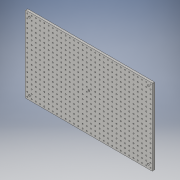
# Autodesk Inventor part: MB1830_solid
Saved by Autodesk Inventor 2016 (Build 200138000, 138)
## iProperties
Created: 2018-01-13
Part Number: MB1830_solid
Material: Generic
Document SubType Name: Modeling
Designer: harveylab
Density: 1 g/cm^3
Appearance: Default
Author: harveylab
Autodesk Inventor part; units mm, degrees
ref_plane "YZ Plane" through (0, 0, 0) normal (1, 0, 0) x (0, 1, 0)
ref_plane "XZ Plane" through (0, 0, 0) normal (0, 1, 0) x (-1, 0, 0)
ref_plane "XY Plane" through (0, 0, 0) normal (0, 0, 1) x (1, 0, 0)
sketch "Sketch1" plane through (0, 0, 0) normal (0, 0, 1) x (1, 0, 0)
  line L0 (-2.7, 453.9) -> (-2.7, 2.7)
  arc A0 (-2.7, 2.7) -> (0, 0) centre (0, 2.7) ccw
  line L1 (0, 0) -> (756, 0)
  arc A1 (756, 0) -> (758.7, 2.7) centre (756, 2.7) ccw
  line L2 (758.7, 2.7) -> (758.7, 453.9)
  arc A2 (758.7, 453.9) -> (756, 456.6) centre (756, 453.9) ccw
  line L3 (756, 456.6) -> (0, 456.6)
  arc A3 (0, 456.6) -> (-2.7, 453.9) centre (0, 453.9) ccw
  circle A4 centre (60.5, 37.8) radius 3.5
  circle A5 centre (85.9, 37.8) radius 3.5
  circle A6 centre (111.3, 37.8) radius 3.5
  circle A7 centre (136.7, 37.8) radius 3.5
  circle A8 centre (162.1, 37.8) radius 3.5
  circle A9 centre (187.5, 37.8) radius 3.5
  circle A10 centre (212.9, 37.8) radius 3.5
  circle A11 centre (238.3, 37.8) radius 3.5
  circle A12 centre (263.7, 37.8) radius 3.5
  circle A13 centre (289.1, 37.8) radius 3.5
  circle A14 centre (314.5, 37.8) radius 3.5
  circle A15 centre (339.9, 37.8) radius 3.5
  circle A16 centre (365.3, 37.8) radius 3.5
  circle A17 centre (390.7, 37.8) radius 3.5
  circle A18 centre (416.1, 37.8) radius 3.5
  circle A19 centre (441.5, 37.8) radius 3.5
  circle A20 centre (466.9, 37.8) radius 3.5
  circle A21 centre (492.3, 37.8) radius 3.5
  circle A22 centre (517.7, 37.8) radius 3.5
  circle A23 centre (543.1, 37.8) radius 3.5
  circle A24 centre (568.5, 37.8) radius 3.5
  circle A25 centre (593.9, 37.8) radius 3.5
  circle A26 centre (619.3, 37.8) radius 3.5
  circle A27 centre (644.7, 37.8) radius 3.5
  circle A28 centre (670.1, 37.8) radius 3.5
  circle A29 centre (695.5, 37.8) radius 3.5
  circle A30 centre (720.9, 37.8) radius 3.5
  circle A31 centre (35.1, 63.2) radius 3.5
  circle A32 centre (60.5, 63.2) radius 3.5
  circle A33 centre (85.9, 63.2) radius 3.5
  circle A34 centre (111.3, 63.2) radius 3.5
  circle A35 centre (136.7, 63.2) radius 3.5
  circle A36 centre (162.1, 63.2) radius 3.5
  circle A37 centre (187.5, 63.2) radius 3.5
  circle A38 centre (212.9, 63.2) radius 3.5
  circle A39 centre (238.3, 63.2) radius 3.5
  circle A40 centre (263.7, 63.2) radius 3.5
  circle A41 centre (289.1, 63.2) radius 3.5
  circle A42 centre (314.5, 63.2) radius 3.5
  circle A43 centre (339.9, 63.2) radius 3.5
  circle A44 centre (365.3, 63.2) radius 3.5
  circle A45 centre (390.7, 63.2) radius 3.5
  circle A46 centre (416.1, 63.2) radius 3.5
  circle A47 centre (441.5, 63.2) radius 3.5
  circle A48 centre (466.9, 63.2) radius 3.5
  circle A49 centre (492.3, 63.2) radius 3.5
  circle A50 centre (517.7, 63.2) radius 3.5
  circle A51 centre (543.1, 63.2) radius 3.5
  circle A52 centre (568.5, 63.2) radius 3.5
  circle A53 centre (593.9, 63.2) radius 3.5
  circle A54 centre (619.3, 63.2) radius 3.5
  circle A55 centre (644.7, 63.2) radius 3.5
  circle A56 centre (670.1, 63.2) radius 3.5
  circle A57 centre (695.5, 63.2) radius 3.5
  circle A58 centre (720.9, 63.2) radius 3.5
  circle A59 centre (35.1, 88.6) radius 3.5
  circle A60 centre (60.5, 88.6) radius 3.5
  circle A61 centre (85.9, 88.6) radius 3.5
  circle A62 centre (111.3, 88.6) radius 3.5
  circle A63 centre (136.7, 88.6) radius 3.5
  circle A64 centre (162.1, 88.6) radius 3.5
  circle A65 centre (187.5, 88.6) radius 3.5
  circle A66 centre (212.9, 88.6) radius 3.5
  circle A67 centre (238.3, 88.6) radius 3.5
  circle A68 centre (263.7, 88.6) radius 3.5
  circle A69 centre (289.1, 88.6) radius 3.5
  circle A70 centre (314.5, 88.6) radius 3.5
  circle A71 centre (339.9, 88.6) radius 3.5
  circle A72 centre (365.3, 88.6) radius 3.5
  circle A73 centre (390.7, 88.6) radius 3.5
  circle A74 centre (416.1, 88.6) radius 3.5
  circle A75 centre (441.5, 88.6) radius 3.5
  circle A76 centre (466.9, 88.6) radius 3.5
  circle A77 centre (492.3, 88.6) radius 3.5
  circle A78 centre (517.7, 88.6) radius 3.5
  circle A79 centre (543.1, 88.6) radius 3.5
  circle A80 centre (568.5, 88.6) radius 3.5
  circle A81 centre (593.9, 88.6) radius 3.5
  circle A82 centre (619.3, 88.6) radius 3.5
  circle A83 centre (644.7, 88.6) radius 3.5
  circle A84 centre (670.1, 88.6) radius 3.5
  circle A85 centre (695.5, 88.6) radius 3.5
  circle A86 centre (720.9, 88.6) radius 3.5
  circle A87 centre (35.1, 114) radius 3.5
  circle A88 centre (60.5, 114) radius 3.5
  circle A89 centre (85.9, 114) radius 3.5
  circle A90 centre (111.3, 114) radius 3.5
  circle A91 centre (136.7, 114) radius 3.5
  circle A92 centre (162.1, 114) radius 3.5
  circle A93 centre (187.5, 114) radius 3.5
  circle A94 centre (212.9, 114) radius 3.5
  circle A95 centre (238.3, 114) radius 3.5
  circle A96 centre (263.7, 114) radius 3.5
  circle A97 centre (289.1, 114) radius 3.5
  circle A98 centre (314.5, 114) radius 3.5
  circle A99 centre (339.9, 114) radius 3.5
  circle A100 centre (365.3, 114) radius 3.5
  circle A101 centre (390.7, 114) radius 3.5
  circle A102 centre (416.1, 114) radius 3.5
  circle A103 centre (441.5, 114) radius 3.5
  circle A104 centre (466.9, 114) radius 3.5
  circle A105 centre (492.3, 114) radius 3.5
  circle A106 centre (517.7, 114) radius 3.5
  circle A107 centre (543.1, 114) radius 3.5
  circle A108 centre (568.5, 114) radius 3.5
  circle A109 centre (593.9, 114) radius 3.5
  circle A110 centre (619.3, 114) radius 3.5
  circle A111 centre (644.7, 114) radius 3.5
  circle A112 centre (670.1, 114) radius 3.5
  circle A113 centre (695.5, 114) radius 3.5
  circle A114 centre (720.9, 114) radius 3.5
  circle A115 centre (35.1, 139.4) radius 3.5
  circle A116 centre (60.5, 139.4) radius 3.5
  circle A117 centre (85.9, 139.4) radius 3.5
  circle A118 centre (111.3, 139.4) radius 3.5
  circle A119 centre (136.7, 139.4) radius 3.5
  circle A120 centre (162.1, 139.4) radius 3.5
  circle A121 centre (187.5, 139.4) radius 3.5
  circle A122 centre (212.9, 139.4) radius 3.5
  circle A123 centre (238.3, 139.4) radius 3.5
  circle A124 centre (263.7, 139.4) radius 3.5
  circle A125 centre (289.1, 139.4) radius 3.5
  circle A126 centre (314.5, 139.4) radius 3.5
  circle A127 centre (339.9, 139.4) radius 3.5
  circle A128 centre (365.3, 139.4) radius 3.5
  circle A129 centre (390.7, 139.4) radius 3.5
  circle A130 centre (416.1, 139.4) radius 3.5
  circle A131 centre (441.5, 139.4) radius 3.5
  circle A132 centre (466.9, 139.4) radius 3.5
  circle A133 centre (492.3, 139.4) radius 3.5
  circle A134 centre (517.7, 139.4) radius 3.5
  circle A135 centre (543.1, 139.4) radius 3.5
  circle A136 centre (568.5, 139.4) radius 3.5
  circle A137 centre (593.9, 139.4) radius 3.5
  circle A138 centre (619.3, 139.4) radius 3.5
  circle A139 centre (644.7, 139.4) radius 3.5
  circle A140 centre (670.1, 139.4) radius 3.5
  circle A141 centre (695.5, 139.4) radius 3.5
  circle A142 centre (720.9, 139.4) radius 3.5
  circle A143 centre (35.1, 164.8) radius 3.5
  circle A144 centre (60.5, 164.8) radius 3.5
  circle A145 centre (85.9, 164.8) radius 3.5
  circle A146 centre (111.3, 164.8) radius 3.5
  circle A147 centre (136.7, 164.8) radius 3.5
  circle A148 centre (162.1, 164.8) radius 3.5
  circle A149 centre (187.5, 164.8) radius 3.5
  circle A150 centre (212.9, 164.8) radius 3.5
  circle A151 centre (238.3, 164.8) radius 3.5
  circle A152 centre (263.7, 164.8) radius 3.5
  circle A153 centre (289.1, 164.8) radius 3.5
  circle A154 centre (314.5, 164.8) radius 3.5
  circle A155 centre (339.9, 164.8) radius 3.5
  circle A156 centre (365.3, 164.8) radius 3.5
  circle A157 centre (390.7, 164.8) radius 3.5
  circle A158 centre (416.1, 164.8) radius 3.5
  circle A159 centre (441.5, 164.8) radius 3.5
  circle A160 centre (466.9, 164.8) radius 3.5
  circle A161 centre (492.3, 164.8) radius 3.5
  circle A162 centre (517.7, 164.8) radius 3.5
  circle A163 centre (543.1, 164.8) radius 3.5
  circle A164 centre (568.5, 164.8) radius 3.5
  circle A165 centre (593.9, 164.8) radius 3.5
  circle A166 centre (619.3, 164.8) radius 3.5
  circle A167 centre (644.7, 164.8) radius 3.5
  circle A168 centre (670.1, 164.8) radius 3.5
  circle A169 centre (695.5, 164.8) radius 3.5
  circle A170 centre (720.9, 164.8) radius 3.5
  circle A171 centre (35.1, 190.2) radius 3.5
  circle A172 centre (60.5, 190.2) radius 3.5
  circle A173 centre (85.9, 190.2) radius 3.5
  circle A174 centre (111.3, 190.2) radius 3.5
  circle A175 centre (136.7, 190.2) radius 3.5
  circle A176 centre (162.1, 190.2) radius 3.5
  circle A177 centre (187.5, 190.2) radius 3.5
  circle A178 centre (212.9, 190.2) radius 3.5
  circle A179 centre (238.3, 190.2) radius 3.5
  circle A180 centre (263.7, 190.2) radius 3.5
  circle A181 centre (289.1, 190.2) radius 3.5
  circle A182 centre (314.5, 190.2) radius 3.5
  circle A183 centre (339.9, 190.2) radius 3.5
  circle A184 centre (365.3, 190.2) radius 3.5
  circle A185 centre (390.7, 190.2) radius 3.5
  circle A186 centre (416.1, 190.2) radius 3.5
  circle A187 centre (441.5, 190.2) radius 3.5
  circle A188 centre (466.9, 190.2) radius 3.5
  circle A189 centre (492.3, 190.2) radius 3.5
  circle A190 centre (517.7, 190.2) radius 3.5
  circle A191 centre (543.1, 190.2) radius 3.5
  circle A192 centre (568.5, 190.2) radius 3.5
  circle A193 centre (593.9, 190.2) radius 3.5
  circle A194 centre (619.3, 190.2) radius 3.5
  circle A195 centre (644.7, 190.2) radius 3.5
  circle A196 centre (670.1, 190.2) radius 3.5
  circle A197 centre (695.5, 190.2) radius 3.5
  circle A198 centre (720.9, 190.2) radius 3.5
  circle A199 centre (35.1, 215.6) radius 3.5
  circle A200 centre (60.5, 215.6) radius 3.5
  circle A201 centre (85.9, 215.6) radius 3.5
  circle A202 centre (111.3, 215.6) radius 3.5
  circle A203 centre (136.7, 215.6) radius 3.5
  circle A204 centre (162.1, 215.6) radius 3.5
  circle A205 centre (187.5, 215.6) radius 3.5
  circle A206 centre (212.9, 215.6) radius 3.5
  circle A207 centre (238.3, 215.6) radius 3.5
  circle A208 centre (263.7, 215.6) radius 3.5
  circle A209 centre (289.1, 215.6) radius 3.5
  circle A210 centre (314.5, 215.6) radius 3.5
  circle A211 centre (339.9, 215.6) radius 3.5
  circle A212 centre (365.3, 215.6) radius 3.5
  circle A213 centre (390.7, 215.6) radius 3.5
  circle A214 centre (416.1, 215.6) radius 3.5
  circle A215 centre (441.5, 215.6) radius 3.5
  circle A216 centre (466.9, 215.6) radius 3.5
  circle A217 centre (492.3, 215.6) radius 3.5
  circle A218 centre (517.7, 215.6) radius 3.5
  circle A219 centre (543.1, 215.6) radius 3.5
  circle A220 centre (568.5, 215.6) radius 3.5
  circle A221 centre (593.9, 215.6) radius 3.5
  circle A222 centre (619.3, 215.6) radius 3.5
  circle A223 centre (644.7, 215.6) radius 3.5
  circle A224 centre (670.1, 215.6) radius 3.5
  circle A225 centre (695.5, 215.6) radius 3.5
  circle A226 centre (720.9, 215.6) radius 3.5
  circle A227 centre (35.1, 241) radius 3.5
  circle A228 centre (60.5, 241) radius 3.5
  circle A229 centre (85.9, 241) radius 3.5
  circle A230 centre (111.3, 241) radius 3.5
  circle A231 centre (136.7, 241) radius 3.5
  circle A232 centre (162.1, 241) radius 3.5
  circle A233 centre (187.5, 241) radius 3.5
  circle A234 centre (212.9, 241) radius 3.5
  circle A235 centre (238.3, 241) radius 3.5
  circle A236 centre (263.7, 241) radius 3.5
  circle A237 centre (289.1, 241) radius 3.5
  circle A238 centre (314.5, 241) radius 3.5
  circle A239 centre (339.9, 241) radius 3.5
  circle A240 centre (365.3, 241) radius 3.5
  circle A241 centre (390.7, 241) radius 3.5
  circle A242 centre (416.1, 241) radius 3.5
  circle A243 centre (441.5, 241) radius 3.5
  circle A244 centre (466.9, 241) radius 3.5
  circle A245 centre (492.3, 241) radius 3.5
  circle A246 centre (517.7, 241) radius 3.5
  circle A247 centre (543.1, 241) radius 3.5
  circle A248 centre (568.5, 241) radius 3.5
  circle A249 centre (593.9, 241) radius 3.5
  circle A250 centre (619.3, 241) radius 3.5
  circle A251 centre (644.7, 241) radius 3.5
  circle A252 centre (670.1, 241) radius 3.5
  circle A253 centre (695.5, 241) radius 3.5
  circle A254 centre (720.9, 241) radius 3.5
  circle A255 centre (35.1, 266.4) radius 3.5
  circle A256 centre (60.5, 266.4) radius 3.5
  circle A257 centre (85.9, 266.4) radius 3.5
  circle A258 centre (111.3, 266.4) radius 3.5
  circle A259 centre (136.7, 266.4) radius 3.5
  circle A260 centre (162.1, 266.4) radius 3.5
  circle A261 centre (187.5, 266.4) radius 3.5
  circle A262 centre (212.9, 266.4) radius 3.5
  circle A263 centre (238.3, 266.4) radius 3.5
  circle A264 centre (263.7, 266.4) radius 3.5
  circle A265 centre (289.1, 266.4) radius 3.5
  circle A266 centre (314.5, 266.4) radius 3.5
  circle A267 centre (339.9, 266.4) radius 3.5
  circle A268 centre (365.3, 266.4) radius 3.5
  circle A269 centre (390.7, 266.4) radius 3.5
  circle A270 centre (416.1, 266.4) radius 3.5
  circle A271 centre (441.5, 266.4) radius 3.5
  circle A272 centre (466.9, 266.4) radius 3.5
  circle A273 centre (492.3, 266.4) radius 3.5
  circle A274 centre (517.7, 266.4) radius 3.5
  circle A275 centre (543.1, 266.4) radius 3.5
  circle A276 centre (568.5, 266.4) radius 3.5
  circle A277 centre (593.9, 266.4) radius 3.5
  circle A278 centre (619.3, 266.4) radius 3.5
  circle A279 centre (644.7, 266.4) radius 3.5
  circle A280 centre (670.1, 266.4) radius 3.5
  circle A281 centre (695.5, 266.4) radius 3.5
  circle A282 centre (720.9, 266.4) radius 3.5
  circle A283 centre (35.1, 291.8) radius 3.5
  circle A284 centre (60.5, 291.8) radius 3.5
  circle A285 centre (85.9, 291.8) radius 3.5
  circle A286 centre (111.3, 291.8) radius 3.5
  circle A287 centre (136.7, 291.8) radius 3.5
  circle A288 centre (162.1, 291.8) radius 3.5
  circle A289 centre (187.5, 291.8) radius 3.5
  circle A290 centre (212.9, 291.8) radius 3.5
  circle A291 centre (238.3, 291.8) radius 3.5
  circle A292 centre (263.7, 291.8) radius 3.5
  circle A293 centre (289.1, 291.8) radius 3.5
  circle A294 centre (314.5, 291.8) radius 3.5
  circle A295 centre (339.9, 291.8) radius 3.5
  circle A296 centre (365.3, 291.8) radius 3.5
  circle A297 centre (390.7, 291.8) radius 3.5
  circle A298 centre (416.1, 291.8) radius 3.5
  circle A299 centre (441.5, 291.8) radius 3.5
  circle A300 centre (466.9, 291.8) radius 3.5
  circle A301 centre (492.3, 291.8) radius 3.5
  circle A302 centre (517.7, 291.8) radius 3.5
  circle A303 centre (543.1, 291.8) radius 3.5
  circle A304 centre (568.5, 291.8) radius 3.5
  circle A305 centre (593.9, 291.8) radius 3.5
  circle A306 centre (619.3, 291.8) radius 3.5
  circle A307 centre (644.7, 291.8) radius 3.5
  circle A308 centre (670.1, 291.8) radius 3.5
  circle A309 centre (695.5, 291.8) radius 3.5
  circle A310 centre (720.9, 291.8) radius 3.5
  circle A311 centre (35.1, 317.2) radius 3.5
  circle A312 centre (60.5, 317.2) radius 3.5
  circle A313 centre (85.9, 317.2) radius 3.5
  circle A314 centre (111.3, 317.2) radius 3.5
  circle A315 centre (136.7, 317.2) radius 3.5
  circle A316 centre (162.1, 317.2) radius 3.5
  circle A317 centre (187.5, 317.2) radius 3.5
  circle A318 centre (212.9, 317.2) radius 3.5
  circle A319 centre (238.3, 317.2) radius 3.5
  circle A320 centre (263.7, 317.2) radius 3.5
  circle A321 centre (289.1, 317.2) radius 3.5
  circle A322 centre (314.5, 317.2) radius 3.5
  circle A323 centre (339.9, 317.2) radius 3.5
  circle A324 centre (365.3, 317.2) radius 3.5
  circle A325 centre (390.7, 317.2) radius 3.5
  circle A326 centre (416.1, 317.2) radius 3.5
  circle A327 centre (441.5, 317.2) radius 3.5
  circle A328 centre (466.9, 317.2) radius 3.5
  circle A329 centre (492.3, 317.2) radius 3.5
  circle A330 centre (517.7, 317.2) radius 3.5
  circle A331 centre (543.1, 317.2) radius 3.5
  circle A332 centre (568.5, 317.2) radius 3.5
  circle A333 centre (593.9, 317.2) radius 3.5
  circle A334 centre (619.3, 317.2) radius 3.5
  circle A335 centre (644.7, 317.2) radius 3.5
  circle A336 centre (670.1, 317.2) radius 3.5
  circle A337 centre (695.5, 317.2) radius 3.5
  circle A338 centre (720.9, 317.2) radius 3.5
  circle A339 centre (35.1, 342.6) radius 3.5
  circle A340 centre (60.5, 342.6) radius 3.5
  circle A341 centre (85.9, 342.6) radius 3.5
  circle A342 centre (111.3, 342.6) radius 3.5
  circle A343 centre (136.7, 342.6) radius 3.5
  circle A344 centre (162.1, 342.6) radius 3.5
  circle A345 centre (187.5, 342.6) radius 3.5
  circle A346 centre (212.9, 342.6) radius 3.5
  circle A347 centre (238.3, 342.6) radius 3.5
  circle A348 centre (263.7, 342.6) radius 3.5
  circle A349 centre (289.1, 342.6) radius 3.5
  circle A350 centre (314.5, 342.6) radius 3.5
  circle A351 centre (339.9, 342.6) radius 3.5
  circle A352 centre (365.3, 342.6) radius 3.5
  circle A353 centre (390.7, 342.6) radius 3.5
  circle A354 centre (416.1, 342.6) radius 3.5
  circle A355 centre (441.5, 342.6) radius 3.5
  circle A356 centre (466.9, 342.6) radius 3.5
  circle A357 centre (492.3, 342.6) radius 3.5
  circle A358 centre (517.7, 342.6) radius 3.5
  circle A359 centre (543.1, 342.6) radius 3.5
  circle A360 centre (568.5, 342.6) radius 3.5
  circle A361 centre (593.9, 342.6) radius 3.5
  circle A362 centre (619.3, 342.6) radius 3.5
  circle A363 centre (644.7, 342.6) radius 3.5
  circle A364 centre (670.1, 342.6) radius 3.5
  circle A365 centre (695.5, 342.6) radius 3.5
  circle A366 centre (720.9, 342.6) radius 3.5
  circle A367 centre (35.1, 368) radius 3.5
  circle A368 centre (60.5, 368) radius 3.5
  circle A369 centre (85.9, 368) radius 3.5
  circle A370 centre (111.3, 368) radius 3.5
  circle A371 centre (136.7, 368) radius 3.5
  circle A372 centre (162.1, 368) radius 3.5
  circle A373 centre (187.5, 368) radius 3.5
  circle A374 centre (212.9, 368) radius 3.5
  circle A375 centre (238.3, 368) radius 3.5
  circle A376 centre (263.7, 368) radius 3.5
  circle A377 centre (289.1, 368) radius 3.5
  circle A378 centre (314.5, 368) radius 3.5
  circle A379 centre (339.9, 368) radius 3.5
  circle A380 centre (365.3, 368) radius 3.5
  circle A381 centre (390.7, 368) radius 3.5
  circle A382 centre (416.1, 368) radius 3.5
  circle A383 centre (441.5, 368) radius 3.5
  circle A384 centre (466.9, 368) radius 3.5
  circle A385 centre (492.3, 368) radius 3.5
  circle A386 centre (517.7, 368) radius 3.5
  circle A387 centre (543.1, 368) radius 3.5
  circle A388 centre (568.5, 368) radius 3.5
  circle A389 centre (593.9, 368) radius 3.5
  circle A390 centre (619.3, 368) radius 3.5
  circle A391 centre (644.7, 368) radius 3.5
  circle A392 centre (670.1, 368) radius 3.5
  circle A393 centre (695.5, 368) radius 3.5
  circle A394 centre (720.9, 368) radius 3.5
  circle A395 centre (35.1, 393.4) radius 3.5
  circle A396 centre (60.5, 393.4) radius 3.5
  circle A397 centre (85.9, 393.4) radius 3.5
  circle A398 centre (111.3, 393.4) radius 3.5
  circle A399 centre (136.7, 393.4) radius 3.5
  circle A400 centre (162.1, 393.4) radius 3.5
  circle A401 centre (187.5, 393.4) radius 3.5
  circle A402 centre (212.9, 393.4) radius 3.5
  circle A403 centre (238.3, 393.4) radius 3.5
  circle A404 centre (263.7, 393.4) radius 3.5
  circle A405 centre (289.1, 393.4) radius 3.5
  circle A406 centre (314.5, 393.4) radius 3.5
  circle A407 centre (339.9, 393.4) radius 3.5
  circle A408 centre (365.3, 393.4) radius 3.5
  circle A409 centre (390.7, 393.4) radius 3.5
  circle A410 centre (416.1, 393.4) radius 3.5
  circle A411 centre (441.5, 393.4) radius 3.5
  circle A412 centre (466.9, 393.4) radius 3.5
  circle A413 centre (492.3, 393.4) radius 3.5
  circle A414 centre (517.7, 393.4) radius 3.5
  circle A415 centre (543.1, 393.4) radius 3.5
  circle A416 centre (568.5, 393.4) radius 3.5
  circle A417 centre (593.9, 393.4) radius 3.5
  circle A418 centre (619.3, 393.4) radius 3.5
  circle A419 centre (644.7, 393.4) radius 3.5
  circle A420 centre (670.1, 393.4) radius 3.5
  circle A421 centre (695.5, 393.4) radius 3.5
  circle A422 centre (720.9, 393.4) radius 3.5
  circle A423 centre (35.1, 418.8) radius 3.5
  circle A424 centre (60.5, 418.8) radius 3.5
  circle A425 centre (85.9, 418.8) radius 3.5
  circle A426 centre (111.3, 418.8) radius 3.5
  circle A427 centre (136.7, 418.8) radius 3.5
  circle A428 centre (162.1, 418.8) radius 3.5
  circle A429 centre (187.5, 418.8) radius 3.5
  circle A430 centre (212.9, 418.8) radius 3.5
  circle A431 centre (238.3, 418.8) radius 3.5
  circle A432 centre (263.7, 418.8) radius 3.5
  circle A433 centre (289.1, 418.8) radius 3.5
  circle A434 centre (314.5, 418.8) radius 3.5
  circle A435 centre (339.9, 418.8) radius 3.5
  circle A436 centre (365.3, 418.8) radius 3.5
  circle A437 centre (390.7, 418.8) radius 3.5
  circle A438 centre (416.1, 418.8) radius 3.5
  circle A439 centre (441.5, 418.8) radius 3.5
  circle A440 centre (466.9, 418.8) radius 3.5
  circle A441 centre (492.3, 418.8) radius 3.5
  circle A442 centre (517.7, 418.8) radius 3.5
  circle A443 centre (543.1, 418.8) radius 3.5
  circle A444 centre (568.5, 418.8) radius 3.5
  circle A445 centre (593.9, 418.8) radius 3.5
  circle A446 centre (619.3, 418.8) radius 3.5
  circle A447 centre (644.7, 418.8) radius 3.5
  circle A448 centre (670.1, 418.8) radius 3.5
  circle A449 centre (695.5, 418.8) radius 3.5
  circle A450 centre (720.9, 418.8) radius 3.5
  circle A451 centre (60.5, 12.4) radius 3.5
  circle A452 centre (85.9, 12.4) radius 3.5
  circle A453 centre (111.3, 12.4) radius 3.5
  circle A454 centre (136.7, 12.4) radius 3.5
  circle A455 centre (162.1, 12.4) radius 3.5
  circle A456 centre (187.5, 12.4) radius 3.5
  circle A457 centre (212.9, 12.4) radius 3.5
  circle A458 centre (238.3, 12.4) radius 3.5
  circle A459 centre (263.7, 12.4) radius 3.5
  circle A460 centre (289.1, 12.4) radius 3.5
  circle A461 centre (314.5, 12.4) radius 3.5
  circle A462 centre (339.9, 12.4) radius 3.5
  circle A463 centre (365.3, 12.4) radius 3.5
  circle A464 centre (390.7, 12.4) radius 3.5
  circle A465 centre (416.1, 12.4) radius 3.5
  circle A466 centre (441.5, 12.4) radius 3.5
  circle A467 centre (466.9, 12.4) radius 3.5
  circle A468 centre (492.3, 12.4) radius 3.5
  circle A469 centre (517.7, 12.4) radius 3.5
  circle A470 centre (543.1, 12.4) radius 3.5
  circle A471 centre (568.5, 12.4) radius 3.5
  circle A472 centre (593.9, 12.4) radius 3.5
  circle A473 centre (619.3, 12.4) radius 3.5
  circle A474 centre (644.7, 12.4) radius 3.5
  circle A475 centre (670.1, 12.4) radius 3.5
  circle A476 centre (695.5, 12.4) radius 3.5
  circle A477 centre (720.9, 12.4) radius 3.5
  circle A478 centre (746.3, 12.4) radius 3.5
  circle A479 centre (9.7, 37.8) radius 3.5
  circle A480 centre (746.3, 37.8) radius 3.5
  circle A481 centre (9.7, 63.2) radius 3.5
  circle A482 centre (746.3, 63.2) radius 3.5
  circle A483 centre (9.7, 88.6) radius 3.5
  circle A484 centre (746.3, 88.6) radius 3.5
  circle A485 centre (9.7, 114) radius 3.5
  circle A486 centre (746.3, 114) radius 3.5
  circle A487 centre (9.7, 139.4) radius 3.5
  circle A488 centre (746.3, 139.4) radius 3.5
  circle A489 centre (9.7, 164.8) radius 3.5
  circle A490 centre (746.3, 164.8) radius 3.5
  circle A491 centre (9.7, 190.2) radius 3.5
  circle A492 centre (746.3, 190.2) radius 3.5
  circle A493 centre (9.7, 215.6) radius 3.5
  circle A494 centre (746.3, 215.6) radius 3.5
  circle A495 centre (9.7, 241) radius 3.5
  circle A496 centre (746.3, 241) radius 3.5
  circle A497 centre (9.7, 266.4) radius 3.5
  circle A498 centre (746.3, 266.4) radius 3.5
  circle A499 centre (9.7, 291.8) radius 3.5
  circle A500 centre (746.3, 291.8) radius 3.5
  circle A501 centre (9.7, 317.2) radius 3.5
  circle A502 centre (746.3, 317.2) radius 3.5
  circle A503 centre (9.7, 342.6) radius 3.5
  circle A504 centre (746.3, 342.6) radius 3.5
  circle A505 centre (9.7, 368) radius 3.5
  circle A506 centre (746.3, 368) radius 3.5
  circle A507 centre (9.7, 393.4) radius 3.5
  circle A508 centre (746.3, 393.4) radius 3.5
  circle A509 centre (9.7, 418.8) radius 3.5
  circle A510 centre (746.3, 418.8) radius 3.5
  circle A511 centre (9.7, 444.2) radius 3.5
  circle A512 centre (35.1, 444.2) radius 3.5
  circle A513 centre (60.5, 444.2) radius 3.5
  circle A514 centre (85.9, 444.2) radius 3.5
  circle A515 centre (111.3, 444.2) radius 3.5
  circle A516 centre (136.7, 444.2) radius 3.5
  circle A517 centre (162.1, 444.2) radius 3.5
  circle A518 centre (187.5, 444.2) radius 3.5
  circle A519 centre (212.9, 444.2) radius 3.5
  circle A520 centre (238.3, 444.2) radius 3.5
  circle A521 centre (263.7, 444.2) radius 3.5
  circle A522 centre (289.1, 444.2) radius 3.5
  circle A523 centre (314.5, 444.2) radius 3.5
  circle A524 centre (339.9, 444.2) radius 3.5
  circle A525 centre (365.3, 444.2) radius 3.5
  circle A526 centre (390.7, 444.2) radius 3.5
  circle A527 centre (416.1, 444.2) radius 3.5
  circle A528 centre (441.5, 444.2) radius 3.5
  circle A529 centre (466.9, 444.2) radius 3.5
  circle A530 centre (492.3, 444.2) radius 3.5
  circle A531 centre (517.7, 444.2) radius 3.5
  circle A532 centre (543.1, 444.2) radius 3.5
  circle A533 centre (568.5, 444.2) radius 3.5
  circle A534 centre (593.9, 444.2) radius 3.5
  circle A535 centre (619.3, 444.2) radius 3.5
  circle A536 centre (644.7, 444.2) radius 3.5
  circle A537 centre (670.1, 444.2) radius 3.5
  circle A538 centre (695.5, 444.2) radius 3.5
  circle A539 centre (720.9, 444.2) radius 3.5
  circle A540 centre (746.3, 444.2) radius 3.5
  circle A541 centre (22.4, 431.5) radius 5.5
  circle A542 centre (733.6, 25.1) radius 5.5
  circle A543 centre (733.6, 431.5) radius 5.5
  circle A544 centre (22.4, 25.1) radius 5.5
  circle A545 centre (378, 228.3) radius 5.5
  circle A546 centre (35.1, 12.4) radius 3.5
  circle A547 centre (35.1, 37.8) radius 3.5
  circle A548 centre (9.7, 12.4) radius 3.5
  point P0 (0, 0)
  constraints: 549 centre point, 8 end point, 8 point on circle, 1 coincident
extrude "Extrusion1" add sketch "Sketch1" along normal blind 12.7
body "Solid1"
